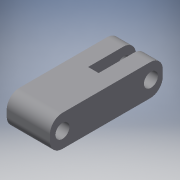
# Autodesk Inventor part: lever2
Saved by Autodesk Inventor 2016 (Build 200138000, 138)
## iProperties
Created: 2015-09-30
Part Number: lever2
Material: Generic
Document SubType Name: Modeling
Designer: Jesse Stevenson
Density: 1 g/cm^3
Appearance: Default
Author: Jesse Stevenson
Autodesk Inventor part; units mm, degrees
ref_plane "YZ Plane" through (0, 0, 0) normal (1, 0, 0) x (0, 1, 0)
ref_plane "XZ Plane" through (0, 0, 0) normal (0, 1, 0) x (-1, 0, 0)
ref_plane "XY Plane" through (0, 0, 0) normal (0, 0, 1) x (1, 0, 0)
ref_plane "Work Plane1" through (8.001, 26.0985, -18.0717) normal (0, 1, 0) x (0, 0, -1)
sketch "Sketch1" plane through (8.001, 26.0985, -18.0717) normal (0, 1, 0) x (0, 0, -1)
  line L0 (-40.2323, -2.2493) -> (-40.2391, -6.3168)
  line L1 (-40.2391, -6.3168) -> (-9.3098, -6.3168)
  line L2 (-9.3098, -6.3168) -> (-9.3098, -4.9466)
  line L3 (-40.2323, 0.3257) -> (-40.2323, 4.3932)
  line L4 (-40.2323, 4.3932) -> (-9.3098, 4.3932)
  line L5 (-9.3098, 4.3932) -> (-9.3098, 3.023)
  line L6 (-40.2323, -2.2493) -> (-40.2323, 0.3257)
  line L7 (-9.3098, -4.9466) -> (-25.0354, -4.9466)
  line L8 (-25.0354, -4.9466) -> (-25.0354, 3.023)
  line L9 (-25.0354, 3.023) -> (-9.3098, 3.023)
  line L10 (-18.0537, -4.9466) -> (-18.0537, -6.3168) construction
  line L11 (-18.0537, 3.023) -> (-18.0537, 4.3932) construction
  line L12 (-17.7595, -4.3116) -> (18.2812, -4.3116) construction
  point P0 (-18.0717, 8.001)
  dimension "d16" = 0.635
  constraints: 24 end point, 6 point on line, 3 parallel, 3 perpendicular, 2 collinear, 2 equal length, 2 horizontal
  measures "d16" distance between parallel lines of L7 L12
extrude "Extrusion1" add sketch "Sketch1" along normal blind 7.9375
sketch "Sketch2" plane through (14.3178, 26.0985, 22.1674) normal (1, 0, 0) x (0, 0, -1)
  line L0 (30.9293, 0) -> (0, 0) construction
  line L1 (30.9293, 0) -> (30.9293, 7.9375) construction
  line L2 (0, 7.9375) -> (30.9293, 7.9375) construction
  line L3 (0, 0) -> (0, 7.9375) construction
  line L4 (30.9293, 0) -> (30.9293, 7.9375) construction
  line L5 (30.9293, 3.9687) -> (0, 3.9687) construction
  line L6 (30.9293, 0) -> (0, 0) construction
  line L7 (25.6796, 0) -> (25.6796, 7.9375) construction
  line L8 (30.9293, 7.9375) -> (14.8298, 7.9375) construction
  circle A0 centre (25.6796, 3.9687) radius 1.7859
  point P0 (22.1674, -26.0985)
  dimension "d8" = 3.5719
  constraints: 4 end point, 3 midpoint, 2 point on line, 1 centre point, 1 perpendicular
  measures "d8" diameter of A0
extrude "Extrusion2" cut sketch "Sketch2" against normal through all
fillet "Fillet1" radius 3.175 3 edges at (12.2841, 34.036, 22.164) (6.9291, 34.036, 22.1606) (12.2841, 26.0985, 22.164)
sketch "Sketch3" plane through (14.3178, 26.0985, -8.7619) normal (1, 0, 0) x (0, 0, -1)
  circle A0 centre (-5.2497, 3.9688) radius 1.7859 projected
  arc A1 (-30.9293, 3.175) -> (-27.7543, 0) centre (-27.6092, 3.175) ccw projected
  line L0 (0, 0) -> (-27.7543, 0) projected
  line L1 (0, 0) -> (0, 7.9375) projected
  line L2 (-27.7543, 7.9375) -> (0, 7.9375) projected
  line L3 (-30.9293, 3.175) -> (-30.9293, 4.7625) projected
  line L4 (-27.6092, 3.175) -> (-27.6092, 4.7625) construction
  circle A2 centre (-27.6092, 3.9687) radius 1.7859
  ellipse E0 centre (-27.7543, 4.7625) end of major axis (-30.9293, 4.7625) minor radius 3.175 (-27.7543, 7.9375) -> (-30.9293, 4.7625) ccw projected
  point P0 (-8.7619, -26.0985)
  dimension "d7" = 3.5719
  constraints: 2 end point, 1 centre point, 1 midpoint, 1 vertical, 2 other
  measures "d7" diameter of A2
extrude "Extrusion3" cut sketch "Sketch3" against normal through all contours A2
sketch "Sketch5" plane through (14.3178, 26.0985, -8.7619) normal (1, 0, 0) x (0, 0, -1)
  circle A0 centre (-27.6092, 3.9688) radius 1.7859 construction
  circle A1 centre (-5.2497, 3.9688) radius 1.7859 construction
  arc A2 (-30.9293, 3.175) -> (-27.7543, 0) centre (-27.6092, 3.175) ccw construction
  line L0 (0, 0) -> (-27.7543, 0) construction
  line L1 (0, 0) -> (0, 7.9375) construction
  line L2 (-27.7543, 7.9375) -> (0, 7.9375) construction
  line L3 (-30.9293, 3.175) -> (-30.9293, 4.7625) construction
  line L4 (-15.9544, 0) -> (0, 0) projected
  line L5 (-2.2351, 0) -> (-2.2351, 7.9375)
  line L6 (-15.9544, 7.9375) -> (0, 7.9375) projected
  line L7 (-2.2351, 0) -> (-8.7527, 0)
  line L8 (-27.7543, 7.9375) -> (0, 7.9375) projected
  line L9 (-2.2351, 0) -> (0, 0)
  line L10 (0, 0) -> (0, 7.9375)
  line L11 (0, 7.9375) -> (-2.2351, 7.9375)
  line L12 (-2.2351, 7.9375) -> (-2.2351, 0)
  ellipse E0 centre (-27.7543, 4.7625) end of major axis (-30.9293, 4.7625) minor radius 3.175 (-27.7543, 7.9375) -> (-30.9293, 4.7625) ccw projected
  point P0 (-8.7619, -26.0985)
  point P1 (-27.8002, 7.9375)
  constraints: 12 end point, 3 point on line, 2 parallel, 2 perpendicular, 1 horizontal, 2 other
extrude "Extrusion4" cut sketch "Sketch5" against normal through all
fillet "Fillet2" radius 3.175 4 edges at (13.6327, 34.036, -6.5269) (4.2929, 34.036, -6.5269) (13.6327, 26.0985, -6.5269) (4.2929, 26.0985, -6.5269)
sketch "Sketch6" plane through (8.001, 26.0985, -18.0717) normal (0, -1, 0) x (1, 0, 0)
  line L0 (3.9988, 46.6729) -> (3.9988, 39.3669) construction
  line L1 (-2.3512, 39.3669) -> (-2.3512, 46.6729) construction
  line L2 (4.6338, 42.6343) -> (4.6338, 39.3486) construction
  line L3 (-2.9862, 39.3486) -> (-2.9862, 42.6343) construction
  line L4 (4.6338, 42.6343) -> (-2.9862, 42.6343)
  line L5 (-2.9862, 42.6343) -> (-2.9862, 31.0791)
  line L6 (-2.9862, 31.0791) -> (4.6338, 31.0791)
  line L7 (4.6338, 31.0791) -> (4.6338, 42.6343)
  point P0 (-8.001, 18.0717)
  dimension "d12" = 0.635
  dimension "d13" = 0.635
  constraints: 12 end point, 4 parallel, 1 horizontal, 1 perpendicular
  measures "d12" distance between parallel lines of L0 L2
  measures "d13" distance between parallel lines of L1 L3
extrude "Extrusion5" cut sketch "Sketch6" against normal through all
body "Solid1"
